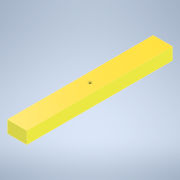
# Autodesk Inventor part: Smiglo
Saved by Autodesk Inventor 2022 (Build 260153000, 153)
## iProperties
Created: 2021-08-09
Part Number: Smiglo
Material: Ogólny
Document SubType Name: Modeling
Designer: Krystyna
Mass: 0.1 g
Surface Area: 16.4785 cm^2
Volume: 2.39804 cm^3
Density: 0.0417008 g/cm^3
Appearance: Lśniąca — złota
Author: Krystyna
Autodesk Inventor part; units mm, degrees
ref_plane "YZ Plane" through (0, 0, 0) normal (1, 0, 0) x (0, 1, 0)
ref_plane "XZ Plane" through (0, 0, 0) normal (0, 1, 0) x (-1, 0, 0)
ref_plane "XY Plane" through (0, 0, 0) normal (0, 0, 1) x (1, 0, 0)
sketch "Szkic1" plane through (0, 0, 0) normal (0, 1, 0) x (-1, 0, 0)
  line L0 (4, 30) -> (-4, 30)
  line L1 (-4, 30) -> (-4, -30)
  line L2 (-4, -30) -> (4, -30)
  line L3 (4, -30) -> (4, 30)
  point P0 (0, 0)
  point P1 (4, 0)
  point P2 (0, -30)
  dimension "d0" = 8
  dimension "d1" = 60
  constraints: 8 end point, 2 midpoint, 2 parallel, 1 horizontal, 1 horizontal alignment, 1 perpendicular, 1 vertical alignment
  measures "d0" distance of L1.end L2.end
  measures "d1" distance of L2.end L0.start
extrude "Wyciągnięcie proste1" add sketch "Szkic1" along normal blind 5
sketch "Szkic2" plane through (0, 5, 0) normal (0, 1, 0) x (1, 0, 0)
  circle A0 centre (0, 0) radius 0.5
  dimension "d4" = 1
  constraints: 1 centre point, 1 coincident
  measures "d4" diameter of A0
extrude "Wyciągnięcie proste2" cut sketch "Szkic2" against normal blind 2.5
